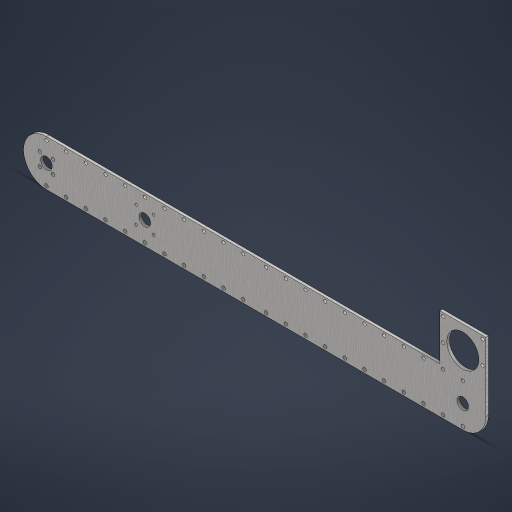
# Autodesk Inventor part: FirstStageArmBar1
Saved by Autodesk Inventor 2024 (Build 280153000, 153)
## iProperties
Created: 2023-11-22
Part Number: FirstStageArmBar1
Material: Generic
Document SubType Name: Modeling
Designer: avsar
Density: 1 g/cm^3
Appearance: Satin Brushed
Author: avsar
Autodesk Inventor part; units mm, degrees
ref_plane "YZ Plane" through (0, 0, 0) normal (1, 0, 0) x (0, 1, 0)
ref_plane "XZ Plane" through (0, 0, 0) normal (0, 1, 0) x (-1, 0, 0)
ref_plane "XY Plane" through (0, 0, 0) normal (0, 0, 1) x (1, 0, 0)
sketch "Sketch1" plane through (0, 0, 0) normal (0, 0, 1) x (1, 0, 0)
  line L0 (-254, -28) -> (254, -28)
  line L1 (282, 0) -> (282, 28)
  line L2 (282, 28) -> (-254, 28) construction
  line L3 (-282, 0) -> (-282, 0)
  line L4 (-282, -28) -> (282, 28) construction
  line L5 (282, -28) -> (-282, 28) construction
  arc A0 (-254, 28) -> (-282, 0) centre (-254, 0) ccw
  arc A1 (-282, 0) -> (-254, -28) centre (-254, 0) ccw
  circle A2 centre (-134, 0) radius 7
  circle A3 centre (-144.6066, 10.6066) radius 1.5
  line L6 (-134, 0) -> (-144.6066, 10.6066) construction
  line L7 (-134, 0) -> (-254, 0) construction
  circle A4 centre (-144.6066, -10.6066) radius 1.5
  circle A5 centre (-123.3934, -10.6066) radius 1.5
  circle A6 centre (-123.3934, 10.6066) radius 1.5
  arc A7 (254, -28) -> (282, 0) centre (254, 0) ccw
  circle A8 centre (254, 0) radius 7
  line L8 (282, 28) -> (282, 84)
  line L9 (282, 84) -> (226, 84)
  line L10 (226, 84) -> (226, 28)
  line L11 (226, 28) -> (-254, 28)
  circle A9 centre (254, 56) radius 19.5
  circle A10 centre (-254, 0) radius 7
  circle A11 centre (-262, 8) radius 2
  circle A12 centre (-262, -8) radius 2
  circle A13 centre (-246, -8) radius 2
  circle A14 centre (-246, 8) radius 2
  point P0 (0, 0)
  point P1 (-282, 0)
  dimension "d1" = 56
  dimension "d3" = 28
  dimension "d4" = 14
  dimension "d5" = 120
  dimension "d6" = 3
  dimension "d7" = 45
  dimension "d8" = 15
  dimension "d11" = 360
  dimension "d13" = 28
  dimension "d16" = 14
  dimension "d17" = 56
  dimension "d18" = 56
  dimension "d19" = 39
  dimension "d20" = 56
  dimension "d21" = 14
  dimension "d22" = 4
  dimension "d23" = 8
  dimension "d24" = 8
  dimension "d27" = 360
  dimension "d49" = 508
  constraints: 24 end point, 15 centre point, 9 point on line, 6 point on circle, 6 tangent, 3 perpendicular, 2 coincident, 2 midpoint, 2 parallel, 1 collinear, 1 concentric, 1 horizontal, 1 horizontal alignment, 1 vertical, 1 vertical alignment, 18 other
  measures "d1" distance of L4.end L5.start
  measures "d3" radius of A0
  measures "d4" diameter of A2
  measures "d5" distance of L6.start L7.end
  measures "d6" diameter of A3
  measures "d7" angle of L7 L6
  measures "d8" distance of L6.start L6.end
  measures "d13" radius of A7
  measures "d16" diameter of A8
  measures "d17" distance of L1.end L8.end
  measures "d18" distance of L8.end L9.end
  measures "d19" diameter of A9
  measures "d20" distance of A9.centre A7.centre
  measures "d21" diameter of A10
  measures "d22" diameter of A11
  measures "d23" horizontal distance of A11.centre L7.end
  measures "d24" horizontal distance of L7.end A11.centre
  measures "d49" distance of A7.centre A0.centre
extrude "Extrusion1" add sketch "Sketch1" along normal blind 3.175
sketch "Sketch2" plane through (0, 0, 3.175) normal (0, 0, 1) x (1, 0, 0)
  line L0 (226, 28) -> (-254, 28) construction
  circle A0 centre (-254, 24) radius 2
  circle A1 centre (-230, 24) radius 2
  circle A2 centre (-206, 24) radius 2
  circle A3 centre (-182, 24) radius 2
  circle A4 centre (-158, 24) radius 2
  circle A5 centre (-134, 24) radius 2
  circle A6 centre (-110, 24) radius 2
  circle A7 centre (-86, 24) radius 2
  circle A8 centre (-62, 24) radius 2
  circle A9 centre (-38, 24) radius 2
  circle A10 centre (-14, 24) radius 2
  line L1 (0, 28) -> (0, -28) construction
  line L2 (-254, -28) -> (254, -28) construction
  circle A11 centre (254, 24) radius 2
  circle A12 centre (230, 24) radius 2
  circle A13 centre (206, 24) radius 2
  circle A14 centre (182, 24) radius 2
  circle A15 centre (158, 24) radius 2
  circle A16 centre (134, 24) radius 2
  circle A17 centre (110, 24) radius 2
  circle A18 centre (86, 24) radius 2
  circle A19 centre (62, 24) radius 2
  circle A20 centre (38, 24) radius 2
  circle A21 centre (14, 24) radius 2
  arc A22 (-254, 28) -> (-254, -28) centre (-254, 0) ccw construction
  arc A23 (254, -28) -> (282, 0) centre (254, 0) ccw construction
  line L3 (-282, 0) -> (282, 0) construction
  line L4 (226, -28) -> (-254, -28) construction
  circle A24 centre (-254, -24) radius 2
  circle A25 centre (-230, -24) radius 2
  circle A26 centre (-206, -24) radius 2
  circle A27 centre (-182, -24) radius 2
  circle A28 centre (-158, -24) radius 2
  circle A29 centre (-134, -24) radius 2
  circle A30 centre (-110, -24) radius 2
  circle A31 centre (-86, -24) radius 2
  circle A32 centre (-62, -24) radius 2
  circle A33 centre (-38, -24) radius 2
  circle A34 centre (-14, -24) radius 2
  circle A35 centre (62, -24) radius 2
  circle A36 centre (38, -24) radius 2
  circle A37 centre (14, -24) radius 2
  circle A38 centre (86, -24) radius 2
  circle A39 centre (110, -24) radius 2
  circle A40 centre (134, -24) radius 2
  circle A41 centre (158, -24) radius 2
  circle A42 centre (182, -24) radius 2
  circle A43 centre (206, -24) radius 2
  circle A44 centre (230, -24) radius 2
  circle A45 centre (254, -24) radius 2
  circle A46 centre (230, 80) radius 2
  line L5 (226, 84) -> (226, 28) construction
  line L6 (282, 84) -> (226, 84) construction
  circle A47 centre (278, 80) radius 2
  line L7 (282, 0) -> (282, 84) construction
  circle A48 centre (230, 52) radius 2
  circle A49 centre (278, 52) radius 2
  point P0 (0, 0)
  point P1 (254, 28)
  dimension "d29" = 4
  dimension "d30" = 4
  dimension "d33" = 24
  dimension "d38" = 4
  dimension "d39" = 4
  dimension "d40" = 4
  dimension "d41" = 4
  dimension "d42" = 4
  dimension "d43" = 4
  dimension "d44" = 4
  dimension "d45" = 28
  dimension "d46" = 4
  constraints: 48 centre point, 35 symmetric about line, 6 end point, 3 vertical alignment, 2 horizontal, 2 point on line, 1 horizontal alignment, 1 midpoint, 1 point on circle, 1 vertical, 53 other
  measures "d29" diameter of A0
  measures "d30" distance of L0.end A0.centre
  measures "d33" distance of A0.centre A1.centre
  measures "d38" diameter of A46
  measures "d39" distance from line of L5 A46.centre
  measures "d40" distance from line of L6 A46.centre
  measures "d41" diameter of A47
  measures "d42" distance from line of L6 A47.centre
  measures "d43" distance from line of L7 A47.centre
  measures "d44" diameter of A48
  measures "d45" distance of A48.centre A46.centre
  measures "d46" diameter of A49
extrude "Extrusion2" cut sketch "Sketch2" against normal through all
equation "\"d3\" = 0.5 * d1"
equation "\"d13\" = d3"
body "Solid1"
